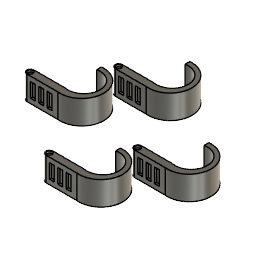
Holder (Autodesk Fusion 360 design; units mm, degrees)
part number: 2026-02-15-21-37-48-238
Autodesk Fusion 360 part; units mm, degrees
sketch "Sketch1" plane through (0, 0, 0) normal (0, 0, 1) x (1, 0, 0)
  line L0 (0, 0) -> (-65, 0)
  line L1 (-69.9513, 3.5481) -> (-69.9513, 3.5474)
  line L2 (0, 15) -> (-65, 15)
  arc A0 (-65, 15) -> (-65, 0) centre (-65, 7.5) ccw
  circle A1 centre (-65, 7.5) radius 5
  line L3 (0, 81) -> (0, 91)
  arc A2 (0, 0) -> (0, 91) centre (4.5, 45.5) ccw
  arc A3 (0, 15) -> (0, 81) centre (6.4375, 48) ccw
  dimension "d41" = 10
  constraint coincident L0.start A2.start
  constraint horizontal L0
  constraint horizontal L2
  constraint tangent L0 A0
  constraint tangent L2 A0
  constraint concentric A0 A1
  measures "d41" diameter of A1
extrude "Extrude1" add sketch "Sketch1" along normal blind 50 contours L0 L2 A0 L3 A2 A3 | A1 makes body 1
ref_plane "WorkPlane1" through (-7.0772, 45.5, 50) normal (0, 0, 1) x (1, 0, 0)
sketch "Sketch2" plane through (0, 0, 50) normal (0, 0, 1) x (1, 0, 0)
  circle A0 centre (-65, 7.5) radius 5.5
  dimension "d52" = 11
  measures "d52" diameter of A0
extrude "Extrude2" cut sketch "Sketch2" against normal blind 4 bodies 1
ref_plane "WorkPlane2" through (-7.0772, 45.5, 0) normal (0, 0, -1) x (-1, 0, 0)
sketch "Sketch3" plane through (0, 0, 0) normal (0, 0, -1) x (-1, 0, 0)
  circle A0 centre (65, 7.5) radius 5.5
  dimension "d53" = 11
  measures "d53" diameter of A0
extrude "Extrude3" cut sketch "Sketch3" against normal blind 4 bodies 1
ref_plane "WorkPlane3" through (-32.5, 0, 25) normal (0, -1, 0) x (1, 0, 0)
sketch "Sketch4" plane through (0, 0, 0) normal (0, -1, 0) x (-1, 0, 0)
  line L0 (0, -50) -> (70, -50)
  line L1 (70, -50) -> (70, 0)
  line L2 (30, -10) -> (40, -10)
  line L3 (40, -10) -> (40, -40)
  line L4 (40, -40) -> (30, -40)
  line L5 (30, -40) -> (30, -10)
  line L6 (30, -10) -> (40, -40) construction
  line L7 (40, -10) -> (30, -40) construction
  line L8 (47.5, -40) -> (57.5, -40)
  line L9 (57.5, -40) -> (57.5, -10)
  line L10 (57.5, -10) -> (47.5, -10)
  line L11 (47.5, -10) -> (47.5, -40)
  line L12 (47.5, -40) -> (57.5, -10) construction
  line L13 (57.5, -40) -> (47.5, -10) construction
  line L14 (22.5, -10) -> (12.5, -10)
  line L15 (12.5, -10) -> (12.5, -40)
  line L16 (12.5, -40) -> (22.5, -40)
  line L17 (22.5, -40) -> (22.5, -10)
  line L18 (22.5, -10) -> (12.5, -40) construction
  line L19 (12.5, -10) -> (22.5, -40) construction
  point P0 (35, -25)
  point P1 (17.5, -25)
  point P2 (52.5, -25)
  point P3 (35, -25)
  point P4 (52.5, -25)
  point P5 (17.5, -25)
  dimension "d33" = 10
  dimension "d35" = 10
  dimension "d36" = 30
  dimension "d37" = 10
  dimension "d38" = 30
  constraint horizontal L0
  constraint perpendicular L0 L1
  constraint horizontal L2
  constraint perpendicular L2 L3
  constraint parallel L2 L4
  constraint parallel L3 L5
  constraint coincident L6 P3
  constraint coincident L7 P3
  constraint coincident P3 P0
  constraint horizontal L8
  constraint perpendicular L8 L9
  constraint parallel L8 L10
  constraint parallel L9 L11
  constraint coincident L12 P4
  constraint coincident L13 P4
  constraint coincident P4 P2
  constraint horizontal L14
  constraint perpendicular L14 L15
  constraint parallel L14 L16
  constraint parallel L15 L17
  constraint coincident L18 P5
  constraint coincident L19 P5
  constraint coincident P1 P5
  measures "d33" distance of L3.end L4.end
  measures "d35" distance of L9.end L10.end
  measures "d36" distance of L8.end L9.end
  measures "d37" distance of L15.end L16.end
  measures "d38" distance of L14.end L15.end
extrude "Extrude4" cut sketch "Sketch4" against normal blind 4.5 bodies 1
copy_body "CopyPasteBodies1" bodies 1 makes body 2
move_body "Move1" bodies 2 to x (1, 0, 0) y (0, 1, 0) z (0, 0, 1) at (68.9191, -29.0748, -97.9939)
copy_body "CopyPasteBodies2" bodies 1 2 makes body 3 makes body 4
move_body "Move2" bodies 3 4 to x (1, 0, 0) y (0, 1, 0) z (0, 0, 1) at (-89.1344, -95.6552, -6.5208)
sketch "Sketch5" plane through (0, -29.0748, 0) normal (0, -1, 0) x (1, 0, 0)
  line L0 (56.4191, -87.9939) -> (46.4191, -87.9939)
  line L1 (46.4191, -87.9939) -> (46.4191, -57.9939)
  line L2 (46.4191, -57.9939) -> (56.4191, -57.9939)
  line L3 (56.4191, -57.9939) -> (56.4191, -87.9939)
  line L4 (28.9191, -87.9939) -> (28.9191, -57.9939)
  line L5 (28.9191, -57.9939) -> (38.9191, -57.9939)
  line L6 (38.9191, -57.9939) -> (38.9191, -87.9939)
  line L7 (38.9191, -87.9939) -> (28.9191, -87.9939)
  line L8 (11.4191, -57.9939) -> (21.4191, -57.9939)
  line L9 (21.4191, -57.9939) -> (21.4191, -87.9939)
  line L10 (21.4191, -87.9939) -> (11.4191, -87.9939)
  line L11 (11.4191, -87.9939) -> (11.4191, -57.9939)
  line L12 (3.9191, -97.9939) -> (68.9191, -97.9939)
  line L13 (68.9191, -47.9939) -> (3.9191, -47.9939)
  line L14 (68.9191, -97.9939) -> (68.9191, -47.9939)
  line L15 (3.9191, -47.9939) -> (3.9191, -97.9939)
